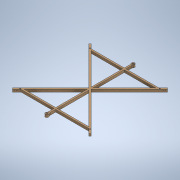
# Autodesk Inventor part: base mesa
Saved by Autodesk Inventor 2022 (Build 260153000, 153)
## iProperties
Created: 2022-02-16
Part Number: base mesa
Material: MDF - Chapa de fibra de média densidade
Document SubType Name: Modeling
Designer: mathe
Density: 0.8 g/cm^3
Appearance: Papelão - Corrugado
Mass: 322.815 g
Surface Area: 1357.05 cm^2
Volume: 403.519 cm^3
Author: mathe
Autodesk Inventor part; units mm, degrees
ref_plane "YZ Plane" through (0, 0, 0) normal (1, 0, 0) x (0, 1, 0)
ref_plane "XZ Plane" through (0, 0, 0) normal (0, 1, 0) x (-1, 0, 0)
ref_plane "XY Plane" through (0, 0, 0) normal (0, 0, 1) x (1, 0, 0)
sketch "Esboço1" plane through (0, 0, 0) normal (0, 1, 0) x (-1, 0, 0)
  line L0 (427.9289, -435) -> (454.7487, -461.8198)
  line L1 (433.5355, -426.4645) -> (461.8198, -454.7487)
  line L2 (433.5355, -3.5355) -> (461.8198, 24.7487)
  line L3 (427.9289, 5) -> (454.7487, 31.8198)
  line L4 (-3.5355, -3.5355) -> (-31.8198, 24.7487)
  line L5 (2.0711, 5) -> (-24.7487, 31.8198)
  line L6 (2.0711, -435) -> (-24.7487, -461.8198)
  line L7 (-3.5355, -426.4645) -> (-31.8198, -454.7487)
  line L8 (2.0711, 5) -> (210, 5)
  line L9 (220, 5) -> (427.9289, 5)
  line L10 (220, -5) -> (417.9289, -5)
  line L11 (220, 40) -> (220, 5)
  line L12 (210, 40) -> (210, 5)
  line L13 (220, -5) -> (220, -202.9289)
  line L14 (12.0711, -5) -> (210, -202.9289)
  line L15 (417.9289, -5) -> (220, -202.9289)
  line L16 (210, -5) -> (210, -202.9289)
  line L17 (207.9289, -215) -> (-3.5355, -426.4645)
  line L18 (-3.5355, -3.5355) -> (207.9289, -215)
  line L19 (220, -227.0711) -> (417.9289, -425)
  line L20 (433.5355, -3.5355) -> (222.0711, -215)
  line L21 (222.0711, -215) -> (433.5355, -426.4645)
  line L22 (210, -227.0711) -> (12.0711, -425)
  line L23 (12.0711, -5) -> (210, -5)
  line L24 (220, -227.0711) -> (220, -425)
  line L25 (220, -435) -> (220, -470)
  line L26 (210, -227.0711) -> (210, -425)
  line L27 (210, -435) -> (210, -470)
  line L28 (417.9289, -425) -> (220, -425)
  line L29 (210, -425) -> (12.0711, -425)
  line L30 (427.9289, -435) -> (220, -435)
  line L31 (210, -435) -> (2.0711, -435)
  arc A0 (220, 55) -> (210, 55) centre (215, 55) ccw
  arc A1 (210, -485) -> (220, -485) centre (215, -485) ccw
  line L32 (-24.7487, -461.8198) -> (-31.8198, -454.7487)
  line L33 (454.7487, -461.8198) -> (461.8198, -454.7487)
  line L34 (454.7487, 31.8198) -> (461.8198, 24.7487)
  line L35 (-24.7487, 31.8198) -> (-31.8198, 24.7487)
  arc A2 (207, -479) -> (223, -479) centre (215, -485) ccw
  circle A3 centre (215, -485) radius 5
  arc A4 (207, -479) -> (210, -470) centre (195, -470) ccw
  arc A5 (220, -470) -> (223, -479) centre (235, -470) ccw
  circle A6 centre (215, -492.5) radius 1.5
  circle A7 centre (222.5, -485) radius 1.5
  circle A8 centre (215, -477.5) radius 1.5
  circle A9 centre (207.5, -485) radius 1.5
  circle A10 centre (215, 55) radius 5
  arc A11 (223, 49) -> (207, 49) centre (215, 55) ccw
  arc A12 (223, 49) -> (220, 40) centre (235, 40) ccw
  arc A13 (210, 40) -> (207, 49) centre (195, 40) ccw
  circle A14 centre (215, 62.5) radius 1.5
  circle A15 centre (207.5, 55) radius 1.5
  circle A16 centre (215, 47.5) radius 1.5
  circle A17 centre (222.5, 55) radius 1.5
  point P0 (0, 0)
  point P1 (220, -476.3397)
  point P2 (210, -476.3397)
  point P3 (220, 46.3397)
  point P4 (210, 46.3397)
  dimension "d75" = 15
  dimension "d76" = 3
  dimension "d79" = 360
  dimension "d81" = 20
  dimension "d82" = 15
  dimension "d83" = 3
  dimension "d86" = 360
  constraints: 72 end point, 20 point on circle, 18 centre point, 8 tangent, 5 coincident, 4 equal radius, 4 point on line, 18 other
  measures "d75" radius of A4
  measures "d76" diameter of A6
  measures "d81" diameter of A11
  measures "d82" radius of A12
  measures "d83" diameter of A14
extrude "Extrusão2" add sketch "Esboço1" along normal blind 15 contours L30 L25 A5 A2 A4 L27 L31 L6 L32 L7 L17 L18 L4 L35 L5 L8 L12 A13 A11 A12 L11 L9 L3 L34 L2 L20 L21 L1 L33 L0 | A10 A0 | A3 A1 | A6 | A7 | A8 | A9 | A14 | A15 | A16 | A17
sketch "Esboço2" plane through (0, 15, 0) normal (0, 1, 0) x (1, 0, 0)
  circle A0 centre (-434.1326, -4.1768) radius 2
  circle A1 centre (4.1504, -4.1768) radius 2
  circle A2 centre (4.1504, 434.0715) radius 2
  circle A3 centre (-434.1326, 434.0715) radius 2
  point P0 (-215, 215)
  point P1 (-215, 215)
  dimension "d33" = 4
  dimension "d34" = 4
  dimension "d35" = 4
  dimension "d36" = 4
  constraints: 4 centre point, 3 coincident
  measures "d33" diameter of A0
  measures "d34" diameter of A1
  measures "d35" diameter of A2
  measures "d36" diameter of A3
extrude "Extrusão3" cut sketch "Esboço2" against normal blind 15
sketch "Esboço3" plane through (0, 15, 0) normal (0, 1, 0) x (1, 0, 0)
  circle A0 centre (4.1504, -4.1768) radius 2 projected
  circle A1 centre (4.1504, -4.1768) radius 3.5
  circle A2 centre (-434.1326, -4.1768) radius 2 projected
  circle A3 centre (-434.1326, -4.1768) radius 3.5
  circle A4 centre (-434.1326, 434.0715) radius 2 projected
  circle A5 centre (-434.1326, 434.0715) radius 3.5
  circle A6 centre (4.1504, 434.0715) radius 2 projected
  circle A7 centre (4.1504, 434.0715) radius 3.5
  point P0 (0, 0)
  dimension "d39" = 7
  dimension "d40" = 7
  dimension "d41" = 7
  dimension "d42" = 7
  constraints: 4 centre point, 4 coincident
  measures "d39" diameter of A1
  measures "d40" diameter of A3
  measures "d41" diameter of A5
  measures "d42" diameter of A7
extrude "Extrusão4" cut sketch "Esboço3" against normal blind 3
sketch "Esboço4" plane through (-207.9289, 0, -215) normal (0.7071068, 0, -0.7071068) x (-0.7071068, 0, -0.7071068)
  line L0 (-339.0559, 0) -> (-339.0559, 15) projected
  line L1 (349.0559, 0) -> (349.0559, 15) projected
  point P0 (-299.0559, 0)
  point P1 (-329.0559, 7.5)
  point P2 (-319.0559, 7.5)
  point P3 (339.0559, 7.5)
  point P4 (329.0559, 7.5)
  dimension "d52" = 10
  dimension "d53" = 10
  dimension "d54" = 10
  dimension "d55" = 10
  measures "d52" distance from line of L0 point (-329.056, 7.5)
  measures "d53" distance of point (-319.056, 7.5) point (-329.056, 7.5)
  measures "d54" distance from line of point (339.056, 7.5) L1
  measures "d55" distance of point (339.056, 7.5) point (329.056, 7.5)
hole "Furo2" at (24.7487, 7.5, 17.6777) at (17.6777, 7.5, 10.6066) at (-447.6777, 7.5, -454.7487) at (-440.6066, 7.5, -447.6777) direction (-0.7071068, 0, 0.7071068) diameter 3 end through all
sketch "Esboço5" plane through (-427.9289, 0, 5) normal (0.7071068, 0, 0.7071068) x (0.7071068, 0, -0.7071068)
  line L0 (-37.9289, 0) -> (-37.9289, 15) projected
  line L1 (650.1829, 0) -> (650.1829, 15) projected
  point P0 (306.127, 0)
  point P1 (-27.9289, 7.5)
  point P2 (-17.9289, 7.5)
  point P3 (640.1829, 7.5)
  point P4 (630.1829, 7.5)
  dimension "d63" = 10
  dimension "d64" = 10
  dimension "d65" = 10
  dimension "d66" = 10
  measures "d63" distance from line of L0 point (-27.929, 7.5)
  measures "d64" distance of point (-27.929, 7.5) point (-17.929, 7.5)
  measures "d65" distance from line of L1 point (640.183, 7.5)
  measures "d66" distance of point (630.183, 7.5) point (640.183, 7.5)
hole "Furo3" at (-447.6777, 7.5, 24.7487) at (-440.6066, 7.5, 17.6777) at (24.7487, 7.5, -447.6777) at (17.6777, 7.5, -440.6066) direction (-0.7071068, 0, -0.7071068) diameter 3 end through all
extrude "Extrusão5" cut sketch "Esboço1" along normal blind 15 contours A10 A0 | A3 A1 | A6 | A7 | A8 | A9 | A14 | A15 | A16 | A17
